Autodesk Inventor part; units mm, degrees
(part 2 of 2)
sketch "Náčrt7" plane through (0, 0, 0) normal (0, 0, -1) x (-1, 0, 0)
  line L0 (-12.458, 1.9719) -> (14.8602, 1.9719) construction
  line L1 (14.8602, 1.9719) -> (14.8602, -1.8119) construction
  line L2 (14.8602, -1.8119) -> (-12.458, -1.8119) construction
  line L3 (-12.458, -1.8119) -> (-12.458, 1.9719) construction
  spline S0 degree 2 poles (-10.9934, -1.8004) (-11.402, -1.8004) (-12.0177, -1.6421) (-12.2824, -1.527) knots 0 0 0 1 2 2 2
  line L4 (-12.2824, -1.527) -> (-12.2824, -0.6811)
  line L5 (-12.2824, -0.6811) -> (-12.2019, -0.6811)
  spline S1 degree 2 poles (-12.2019, -0.6811) (-11.9343, -0.9084) (-11.2926, -1.153) (-10.9905, -1.153) knots 0 0 0 1 2 2 2
  spline S2 degree 2 poles (-10.9905, -1.153) (-10.9128, -1.153) (-10.6625, -1.1184) (-10.5876, -1.0839) knots 0 0 0 1 2 2 2
  spline S3 degree 2 poles (-10.5876, -1.0839) (-10.4956, -1.0436) (-10.3661, -0.8969) (-10.3661, -0.7789) knots 0 0 0 1 2 2 2
  spline S4 degree 2 poles (-10.3661, -0.7789) (-10.3661, -0.6437) (-10.5761, -0.4768) (-10.72, -0.4394) knots 0 0 0 1 2 2 2
  spline S5 degree 2 poles (-10.72, -0.4394) (-10.9013, -0.3905) (-11.3128, -0.307) (-11.494, -0.2437) knots 0 0 0 1 2 2 2
  spline S6 degree 2 poles (-11.494, -0.2437) (-11.9055, -0.0998) (-12.2623, 0.3922) (-12.2623, 0.7605) knots 0 0 0 1 2 2 2
  spline S7 degree 2 poles (-12.2623, 0.7605) (-12.2623, 1.2583) (-11.4192, 1.8769) (-10.7862, 1.8769) knots 0 0 0 1 2 2 2
  spline S8 degree 2 poles (-10.7862, 1.8769) (-10.4697, 1.8769) (-9.8424, 1.7475) (-9.5949, 1.6381) knots 0 0 0 1 2 2 2
  line L6 (-9.5949, 1.6381) -> (-9.5949, 0.8267)
  line L7 (-9.5949, 0.8267) -> (-9.6726, 0.8267)
  spline S9 degree 2 poles (-9.6726, 0.8267) (-9.8712, 0.9965) (-10.4409, 1.2295) (-10.7401, 1.2295) knots 0 0 0 1 2 2 2
  spline S10 degree 2 poles (-10.7401, 1.2295) (-10.8581, 1.2295) (-11.0423, 1.195) (-11.1459, 1.149) knots 0 0 0 1 2 2 2
  spline S11 degree 2 poles (-11.1459, 1.149) (-11.2293, 1.1116) (-11.3502, 0.9619) (-11.3502, 0.8698) knots 0 0 0 1 2 2 2
  spline S12 degree 2 poles (-11.3502, 0.8698) (-11.3502, 0.7317) (-11.1574, 0.5735) (-10.8811, 0.5102) knots 0 0 0 1 2 2 2
  spline S13 degree 2 poles (-10.8811, 0.5102) (-10.7027, 0.4699) (-10.3718, 0.3922) (-10.1819, 0.326) knots 0 0 0 1 2 2 2
  spline S14 degree 2 poles (-10.1819, 0.326) (-9.8136, 0.1908) (-9.4539, -0.2581) (-9.4539, -0.6264) knots 0 0 0 1 2 2 2
  spline S15 degree 2 poles (-9.4539, -0.6264) (-9.4539, -1.1558) (-10.2855, -1.8004) (-10.9934, -1.8004) knots 0 0 0 1 2 2 2
  line L8 (-5.3709, -1.7371) -> (-6.2571, -1.7371)
  line L9 (-6.2571, -1.7371) -> (-6.2571, 0.6166)
  line L10 (-6.2571, 0.6166) -> (-6.9017, -0.9026)
  line L11 (-6.9017, -0.9026) -> (-7.5117, -0.9026)
  line L12 (-7.5117, -0.9026) -> (-8.1562, 0.6166)
  line L13 (-8.1562, 0.6166) -> (-8.1562, -1.7371)
  line L14 (-8.1562, -1.7371) -> (-8.9964, -1.7371)
  line L15 (-8.9964, -1.7371) -> (-8.9964, 1.8136)
  line L16 (-8.9964, 1.8136) -> (-7.9692, 1.8136)
  line L17 (-7.9692, 1.8136) -> (-7.1808, 0.0613)
  line L18 (-7.1808, 0.0613) -> (-6.3981, 1.8136)
  line L19 (-6.3981, 1.8136) -> (-5.3709, 1.8136)
  line L20 (-5.3709, 1.8136) -> (-5.3709, -1.7371)
  line L21 (-5.017, -1.7371) -> (-3.8171, 1.8136)
  line L22 (-3.8171, 1.8136) -> (-2.8445, 1.8136)
  line L23 (-2.8445, 1.8136) -> (-1.6447, -1.7371)
  line L24 (-1.6447, -1.7371) -> (-2.5625, -1.7371)
  line L25 (-2.5625, -1.7371) -> (-2.7841, -1.012)
  line L26 (-2.7841, -1.012) -> (-3.9005, -1.012)
  line L27 (-3.9005, -1.012) -> (-4.125, -1.7371)
  line L28 (-4.125, -1.7371) -> (-5.017, -1.7371)
  line L29 (-2.9798, -0.3674) -> (-3.3423, 0.8065)
  line L30 (-3.3423, 0.8065) -> (-3.7078, -0.3674)
  line L31 (-3.7078, -0.3674) -> (-2.9798, -0.3674)
  line L32 (1.9895, -1.7371) -> (0.9047, -1.7371)
  line L33 (0.9047, -1.7371) -> (-0.0822, -0.4336)
  line L34 (-0.0822, -0.4336) -> (-0.4045, -0.4336)
  line L35 (-0.4045, -0.4336) -> (-0.4045, -1.7371)
  line L36 (-0.4045, -1.7371) -> (-1.2907, -1.7371)
  line L37 (-1.2907, -1.7371) -> (-1.2907, 1.8136)
  line L38 (-1.2907, 1.8136) -> (0.1365, 1.8136)
  spline S16 degree 2 poles (0.1365, 1.8136) (0.4328, 1.8136) (0.8702, 1.7388) (1.0572, 1.6237) knots 0 0 0 1 2 2 2
  spline S17 degree 2 poles (1.0572, 1.6237) (1.2471, 1.5029) (1.4716, 1.1259) (1.4716, 0.8382) knots 0 0 0 1 2 2 2
  spline S18 degree 2 poles (1.4716, 0.8382) (1.4716, 0.4325) (1.1033, -0.0768) (0.7954, -0.2264) knots 0 0 0 1 2 2 2
  line L39 (0.7954, -0.2264) -> (1.9895, -1.7371)
  spline S19 degree 2 poles (0.5566, 0.726) (0.5566, 0.8612) (0.453, 1.054) (0.335, 1.1058) knots 0 0 0 1 2 2 2
  spline S20 degree 2 poles (0.335, 1.1058) (0.2516, 1.1403) (0.0473, 1.1605) (-0.1052, 1.1605) knots 0 0 0 1 2 2 2
  line L40 (-0.1052, 1.1605) -> (-0.4045, 1.1605)
  line L41 (-0.4045, 1.1605) -> (-0.4045, 0.2052)
  line L42 (-0.4045, 0.2052) -> (-0.1484, 0.2052)
  spline S21 degree 2 poles (-0.1484, 0.2052) (0.0358, 0.2052) (0.2976, 0.2512) (0.3868, 0.3231) knots 0 0 0 1 2 2 2
  spline S22 degree 2 poles (0.3868, 0.3231) (0.4731, 0.3922) (0.5566, 0.5764) (0.5566, 0.726) knots 0 0 0 1 2 2 2
  line L43 (2.9362, -1.7371) -> (2.9362, 1.1374)
  line L44 (2.9362, 1.1374) -> (1.8859, 1.1374)
  line L45 (1.8859, 1.1374) -> (1.8859, 1.8136)
  line L46 (1.8859, 1.8136) -> (4.8784, 1.8136)
  line L47 (4.8784, 1.8136) -> (4.8784, 1.1374)
  line L48 (4.8784, 1.1374) -> (3.8282, 1.1374)
  line L49 (3.8282, 1.1374) -> (3.8282, -1.7371)
  line L50 (3.8282, -1.7371) -> (2.9362, -1.7371)
  spline S23 degree 2 poles (6.2625, -1.7975) (5.9862, -1.7975) (5.5287, -1.6277) (5.3647, -1.4551) knots 0 0 0 1 2 2 2
  spline S24 degree 2 poles (5.3647, -1.4551) (5.2007, -1.2853) (5.0194, -0.7616) (5.0194, -0.4106) knots 0 0 0 1 2 2 2
  spline S25 degree 2 poles (5.0194, -0.4106) (5.0194, -0.0596) (5.2065, 0.4526) (5.3647, 0.6253) knots 0 0 0 1 2 2 2
  spline S26 degree 2 poles (5.3647, 0.6253) (5.523, 0.8008) (5.992, 0.9878) (6.2625, 0.9878) knots 0 0 0 1 2 2 2
  spline S27 degree 2 poles (6.2625, 0.9878) (6.4812, 0.9878) (6.8897, 0.8641) (7.048, 0.7835) knots 0 0 0 1 2 2 2
  line L51 (7.048, 0.7835) -> (7.048, 0.28)
  line L52 (7.048, 0.28) -> (7.0221, 0.28)
  spline S28 degree 2 poles (7.0221, 0.28) (6.9732, 0.3203) (6.8236, 0.4238) (6.7171, 0.4785) knots 0 0 0 1 2 2 2
  spline S29 degree 2 poles (6.7171, 0.4785) (6.6221, 0.5246) (6.3689, 0.5965) (6.2538, 0.5965) knots 0 0 0 1 2 2 2
  spline S30 degree 2 poles (6.2538, 0.5965) (5.9057, 0.5965) (5.4827, 0.0699) (5.4827, -0.4106) knots 0 0 0 1 2 2 2
  spline S31 degree 2 poles (5.4827, -0.4106) (5.4827, -0.8796) (5.8913, -1.4062) (6.2538, -1.4062) knots 0 0 0 1 2 2 2
  spline S32 degree 2 poles (6.2538, -1.4062) (6.4725, -1.4062) (6.8696, -1.2249) (7.0221, -1.0839) knots 0 0 0 1 2 2 2
  line L53 (7.0221, -1.0839) -> (7.048, -1.0839)
  line L54 (7.048, -1.0839) -> (7.048, -1.5875)
  spline S33 degree 2 poles (7.048, -1.5875) (6.9818, -1.6191) (6.7804, -1.7083) (6.6998, -1.7285) knots 0 0 0 1 2 2 2
  spline S34 degree 2 poles (6.6998, -1.7285) (6.5847, -1.763) (6.4035, -1.7975) (6.2625, -1.7975) knots 0 0 0 1 2 2 2
  spline S35 degree 2 poles (8.9413, -1.4551) (8.8867, -1.4954) (8.7025, -1.6393) (8.6162, -1.6824) knots 0 0 0 1 2 2 2
  spline S36 degree 2 poles (8.6162, -1.6824) (8.4982, -1.7457) (8.2767, -1.8119) (8.0752, -1.8119) knots 0 0 0 1 2 2 2
  spline S37 degree 2 poles (8.0752, -1.8119) (7.9112, -1.8119) (7.6149, -1.6882) (7.5026, -1.576) knots 0 0 0 1 2 2 2
  spline S38 degree 2 poles (7.5026, -1.576) (7.3962, -1.4666) (7.2667, -1.1443) (7.2667, -0.9659) knots 0 0 0 1 2 2 2
  spline S39 degree 2 poles (7.2667, -0.9659) (7.2667, -0.6897) (7.4998, -0.2984) (7.753, -0.1862) knots 0 0 0 1 2 2 2
  spline S40 degree 2 poles (7.753, -0.1862) (7.9774, -0.0826) (8.5874, -0.0049) (8.9413, 0.0153) knots 0 0 0 1 2 2 2
  line L55 (8.9413, 0.0153) -> (8.9413, 0.1016)
  spline S41 degree 2 poles (8.9413, 0.1016) (8.9413, 0.257) (8.8464, 0.4497) (8.7601, 0.5044) knots 0 0 0 1 2 2 2
  spline S42 degree 2 poles (8.7601, 0.5044) (8.6737, 0.5591) (8.4263, 0.5936) (8.2939, 0.5936) knots 0 0 0 1 2 2 2
  spline S43 degree 2 poles (8.2939, 0.5936) (8.1385, 0.5936) (7.7184, 0.5015) (7.5084, 0.4123) knots 0 0 0 1 2 2 2
  line L56 (7.5084, 0.4123) -> (7.4825, 0.4123)
  line L57 (7.4825, 0.4123) -> (7.4825, 0.8698)
  spline S44 degree 2 poles (7.4825, 0.8698) (7.6062, 0.9044) (8.0695, 0.9907) (8.2968, 0.9907) knots 0 0 0 1 2 2 2
  spline S45 degree 2 poles (8.2968, 0.9907) (8.573, 0.9907) (8.95, 0.9044) (9.0996, 0.7922) knots 0 0 0 1 2 2 2
  spline S46 degree 2 poles (9.0996, 0.7922) (9.2463, 0.6828) (9.3902, 0.3346) (9.3902, 0.0843) knots 0 0 0 1 2 2 2
  line L58 (9.3902, 0.0843) -> (9.3902, -1.7371)
  line L59 (9.3902, -1.7371) -> (8.9413, -1.7371)
  line L60 (8.9413, -1.7371) -> (8.9413, -1.4551)
  line L61 (8.9413, -1.081) -> (8.9413, -0.3415)
  spline S47 degree 2 poles (8.9413, -0.3415) (8.7802, -0.3559) (8.2939, -0.4048) (8.1414, -0.4509) knots 0 0 0 1 2 2 2
  spline S48 degree 2 poles (8.1414, -0.4509) (7.963, -0.5056) (7.73, -0.7329) (7.73, -0.9343) knots 0 0 0 1 2 2 2
  spline S49 degree 2 poles (7.73, -0.9343) (7.73, -1.1645) (7.9889, -1.3976) (8.2364, -1.3976) knots 0 0 0 1 2 2 2
  spline S50 degree 2 poles (8.2364, -1.3976) (8.4464, -1.3976) (8.7917, -1.2163) (8.9413, -1.081) knots 0 0 0 1 2 2 2
  line L62 (11.4332, 0.4469) -> (11.4102, 0.4469)
  spline S51 degree 2 poles (11.4102, 0.4469) (11.3584, 0.4613) (11.2461, 0.467) (11.1685, 0.467) knots 0 0 0 1 2 2 2
  spline S52 degree 2 poles (11.1685, 0.467) (10.9872, 0.467) (10.6304, 0.3088) (10.4692, 0.1534) knots 0 0 0 1 2 2 2
  line L63 (10.4692, 0.1534) -> (10.4692, -1.7371)
  line L64 (10.4692, -1.7371) -> (10.0204, -1.7371)
  line L65 (10.0204, -1.7371) -> (10.0204, 0.9274)
  line L66 (10.0204, 0.9274) -> (10.4692, 0.9274)
  line L67 (10.4692, 0.9274) -> (10.4692, 0.5303)
  spline S53 degree 2 poles (10.4692, 0.5303) (10.7138, 0.749) (11.0793, 0.9274) (11.2519, 0.9274) knots 0 0 0 1 2 2 2
  spline S54 degree 2 poles (11.2519, 0.9274) (11.321, 0.9274) (11.39, 0.9216) (11.4332, 0.913) knots 0 0 0 1 2 2 2
  line L68 (11.4332, 0.913) -> (11.4332, 0.4469)
  line L69 (13.8301, -1.7371) -> (13.3812, -1.7371)
  line L70 (13.3812, -1.7371) -> (13.3812, -1.4666)
  spline S55 degree 2 poles (13.3812, -1.4666) (13.2776, -1.5529) (13.1251, -1.668) (13.0215, -1.7169) knots 0 0 0 1 2 2 2
  spline S56 degree 2 poles (13.0215, -1.7169) (12.9266, -1.763) (12.7223, -1.8119) (12.587, -1.8119) knots 0 0 0 1 2 2 2
  spline S57 degree 2 poles (12.587, -1.8119) (12.3683, -1.8119) (12, -1.6306) (11.8705, -1.4551) knots 0 0 0 1 2 2 2
  spline S58 degree 2 poles (11.8705, -1.4551) (11.7411, -1.2796) (11.5972, -0.7616) (11.5972, -0.425) knots 0 0 0 1 2 2 2
  spline S59 degree 2 poles (11.5972, -0.425) (11.5972, -0.0739) (11.7785, 0.4382) (11.9367, 0.631) knots 0 0 0 1 2 2 2
  spline S60 degree 2 poles (11.9367, 0.631) (12.0835, 0.8037) (12.4949, 1.0022) (12.7223, 1.0022) knots 0 0 0 1 2 2 2
  spline S61 degree 2 poles (12.7223, 1.0022) (12.9208, 1.0022) (13.2172, 0.913) (13.3812, 0.8209) knots 0 0 0 1 2 2 2
  line L71 (13.3812, 0.8209) -> (13.3812, 1.9719)
  line L72 (13.3812, 1.9719) -> (13.8301, 1.9719)
  line L73 (13.8301, 1.9719) -> (13.8301, -1.7371)
  line L74 (13.3812, -1.0897) -> (13.3812, 0.4497)
  spline S62 degree 2 poles (13.3812, 0.4497) (13.2143, 0.5303) (12.9496, 0.5907) (12.7971, 0.5907) knots 0 0 0 1 2 2 2
  spline S63 degree 2 poles (12.7971, 0.5907) (12.4518, 0.5907) (12.0605, 0.0728) (12.0605, -0.4164) knots 0 0 0 1 2 2 2
  spline S64 degree 2 poles (12.0605, -0.4164) (12.0605, -0.8883) (12.3597, -1.386) (12.6906, -1.386) knots 0 0 0 1 2 2 2
  spline S65 degree 2 poles (12.6906, -1.386) (12.8661, -1.386) (13.2229, -1.2249) (13.3812, -1.0897) knots 0 0 0 1 2 2 2
  point P0 (0, 0)
  constraints: 2 other
emboss "Reliéf2" sketch "Náčrt7" operation add depth 0.01 direction (0, 0, 1)
